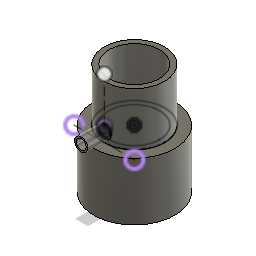
Adapter Validation Lung to 15mm (Autodesk Fusion 360 design; units mm, degrees)
Autodesk Fusion 360 part; units mm, degrees
sketch "Sketch1" plane through (0, 0, 0) normal (0, 1, 0) x (1, 0, 0)
  circle A0 centre (0, 0) radius 12.25
  circle A1 centre (0, 0) radius 10.75
  dimension "d1" = 24.5
  dimension "d2" = 1.5
  constraint coincident A0.centre A1.centre
  constraint concentric A0 A1
  measures "d1" diameter of A0
  measures "d2" distance of A0 A1
extrude "Extrude1" add sketch "Sketch1" along normal blind 16 makes body 1
ref_plane "WorkPlane1" through (0, 16, 0) normal (0, 1, 0) x (1, 0, 0)
sketch "Sketch2" plane through (0, 16, 0) normal (0, 1, 0) x (1, 0, 0)
  circle A0 centre (0, 0) radius 12.25
  circle A1 centre (0, 0) radius 12.25
  constraint coincident A0.centre A1.centre
  constraint tangent A0 A1
extrude "Extrude2" add sketch "Sketch2" along normal blind 1.5 bodies 1
ref_plane "WorkPlane2" through (0, 17.5, 0) normal (0, 1, 0) x (1, 0, 0)
sketch "Sketch3" plane through (0, 17.5, 0) normal (0, 1, 0) x (1, 0, 0)
  circle A0 centre (0, 0) radius 7.6
  circle A1 centre (0, 0) radius 9.1
  dimension "d9" = 15.2
  dimension "d10" = 1.5
  constraint coincident A0.centre A1.centre
  measures "d9" diameter of A0
  measures "d10" distance of A0 A1
extrude "Extrude4" add sketch "Sketch3" along normal blind 16 bodies 1
extrude "Extrude3" cut sketch "Sketch3" against normal blind 1.5 contours A0 bodies 1
ref_plane "WorkPlane3" through (0, 21.8424, 9.1) normal (0, 0, 1) x (-1, 0, 0)
sketch "Sketch4" plane through (0, 21.8424, 9.1) normal (0, 0, 1) x (1, 0, 0)
  circle A0 centre (0, -1.3424) radius 2
  circle A1 centre (0, -1.3424) radius 1.5
  line L0 (0, 0) -> (0, 13.5992) construction
  line L1 (9.1, -4.3424) -> (-9.1, -4.3424) construction
  dimension "d16" = 4
  dimension "d17" = 0.5
  dimension "d18" = 3
  constraint concentric A0 A1
  constraint coincident L0.start origin
  constraint vertical L0
  constraint coincident A0.centre L0
  measures "d16" diameter of A0
  measures "d17" distance of A0 A1
  measures "d18" distance of A0.centre L1
extrude "Extrude6" add sketch "Sketch4" along normal blind 7 bodies 1
extrude "Extrude5" cut sketch "Sketch4" along normal mid plane 10 contours A1 bodies 1
copy_body "Body->Comp1" bodies 1 removing the originals makes body 2 in component "Adapter"
component "Adapter" placed x (1, 0, 0) y (0, 1, 0) z (0, 0, 1) at (0, 0, 0)
